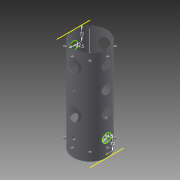
# Autodesk Inventor part: Probe Region Shield
Saved by Autodesk Inventor 2015 (Build 190159000, 159)
## iProperties
Created: 2014-06-23
Part Number: Probe Region Shield
Material: Generic
Document SubType Name: Modeling
Designer: Aki
Density: 1 g/cm^3
Appearance: Default
Author: Aki
Autodesk Inventor part; units mm, degrees
sketch "Sketch1" plane through (0, 0, 0) normal (0, 1, 0) x (-1, 0, 0)
  circle A0 centre (0, 0) radius 84.5
  circle A1 centre (0, 0) radius 85.5
  dimension "d0" = 169
  dimension "d1" = 171
  constraints: 2 centre point, 2 coincident
  measures "d0" diameter of A0
  measures "d1" diameter of A1
extrude "Extrusion1" add sketch "Sketch1" along normal blind 466.5 and the other way blind 15.989
ref_plane "Work Plane1" through (85.5, 0, 0) normal (1, 0, 0) x (0, 1, 0)
ref_plane "Work Plane2" through (-85.5, 0, 0) normal (1, 0, 0) x (0, 1, 0)
sketch "Sketch2" plane through (85.5, 0, 0) normal (1, 0, 0) x (0, 1, 0)
  circle A0 centre (394.5, 0) radius 23.25
  line L0 (466.5, -85.5) -> (466.5, 85.5) projected
  line L1 (-15.989, 85.5) -> (-15.989, -85.5) projected
  point P0 (0, 0)
  dimension "d9" = 46.5
  dimension "d12" = 72
  constraints: 1 centre point, 1 other
  measures "d9" diameter of A0
  measures "d12" distance from line of L0 A0.centre
hole "Hole1" at (85.5, 394.5, 0) direction (-1, 0, 0) diameter 46.5 end through all
sketch "Sketch3" plane through (85.5, 0, 0) normal (1, 0, 0) x (0, 1, 0)
  circle A0 centre (72, 0) radius 23.25
  line L0 (-15.989, 85.5) -> (-15.989, -85.5) projected
  point P0 (0, 0)
  dimension "d21" = 46.5
  dimension "d60" = 72
  constraints: 1 centre point, 1 other
  measures "d21" diameter of A0
  measures "d60" distance of A0.centre point (0, 0)
hole "Hole2" at (85.5, 72, 0) direction (-1, 0, 0) diameter 46.5 end through all
sketch "Sketch4" plane through (85.5, 0, 0) normal (1, 0, 0) x (0, 1, 0)
  circle A0 centre (179.5, 0) radius 23.25
  line L0 (-15.989, 85.5) -> (-15.989, -85.5) projected
  point P0 (0, 0)
  dimension "d30" = 46.5
  dimension "d61" = 179.5
  constraints: 1 centre point, 1 other
  measures "d30" diameter of A0
  measures "d61" distance of A0.centre point (0, 0)
hole "Hole3" at (85.5, 179.5, 0) direction (-1, 0, 0) diameter 46.5 end through all
sketch "Sketch5" plane through (85.5, 0, 0) normal (1, 0, 0) x (0, 1, 0)
  circle A0 centre (287, 0) radius 23.25
  line L0 (-15.989, 85.5) -> (-15.989, -85.5) projected
  point P0 (0, 0)
  dimension "d39" = 46.5
  dimension "d62" = 287
  constraints: 1 centre point, 1 other
  measures "d39" diameter of A0
  measures "d62" distance of A0.centre point (0, 0)
hole "Hole4" at (85.5, 287, 0) direction (-1, 0, 0) diameter 46.5 end through all
sketch "Sketch6" plane through (85.5, 0, 0) normal (1, 0, 0) x (0, 1, 0)
  circle A0 centre (72, 0) radius 22.25
  line L0 (-15.989, 85.5) -> (-15.989, -85.5) projected
  point P0 (0, 0)
  dimension "d48" = 44.5
  dimension "d63" = 72
  constraints: 1 centre point, 1 other
  measures "d48" diameter of A0
  measures "d63" distance of point (0, 0) A0.centre
ref_plane "Work Plane4" through (0, 0, -85.5) normal (0, 0, 1) x (1, 0, 0)
sketch "Sketch9" plane through (0, 0, -85.5) normal (0, 0, 1) x (1, 0, 0)
  circle A0 centre (0, 394.5) radius 35.25
  line L0 (85.5, 466.5) -> (-85.5, 466.5) projected
  point P0 (0, 0)
  dimension "d65" = 70.5
  dimension "d68" = 72
  constraints: 1 centre point
  measures "d65" diameter of A0
  measures "d68" distance from line of L0 A0.centre
sketch "Sketch10" plane through (-85.5, 0, 0) normal (1, 0, 0) x (0, 1, 0)
  circle A0 centre (394.5, 0) radius 22.25
  line L0 (466.5, -85.5) -> (466.5, 85.5) projected
  point P0 (0, 0)
  dimension "d66" = 44.5
  dimension "d67" = 72
  constraints: 1 centre point
  measures "d66" diameter of A0
  measures "d67" distance from line of L0 A0.centre
sketch "Sketch11" plane through (0, 0, -85.5) normal (0, 0, 1) x (1, 0, 0)
  circle A0 centre (0, 179.5) radius 35.25
  line L0 (85.5, 466.5) -> (-85.5, 466.5) projected
  point P0 (0, 0)
  dimension "d69" = 70.5
  dimension "d70" = 287
  constraints: 1 centre point
  measures "d69" diameter of A0
  measures "d70" distance from line of L0 A0.centre
sketch "Sketch12" plane through (0, 0, -85.5) normal (0, 0, 1) x (1, 0, 0)
  circle A0 centre (0, 287) radius 9.9
  line L0 (85.5, 466.5) -> (-85.5, 466.5) projected
  point P0 (0, 0)
  dimension "d71" = 19.8
  dimension "d72" = 179.5
  constraints: 1 centre point
  measures "d71" diameter of A0
  measures "d72" distance from line of L0 A0.centre
sketch "Sketch13" plane through (0, 0, -85.5) normal (0, 0, 1) x (1, 0, 0)
  circle A0 centre (0, 72) radius 9.9
  line L0 (85.5, 466.5) -> (-85.5, 466.5) projected
  point P0 (0, 0)
  dimension "d73" = 19.8
  dimension "d74" = 394.5
  constraints: 1 centre point
  measures "d73" diameter of A0
  measures "d74" distance from line of L0 A0.centre
hole "Hole5" at (0, 394.5, -85.5) direction (0, 0, 1) diameter 70.5 end through all
hole "Hole6" at (0, 179.5, -85.5) direction (0, 0, 1) diameter 70.5 end through all
hole "Hole7" at (0, 287, -85.5) direction (0, 0, 1) diameter 19.8 end through all
hole "Hole8" at (0, 72, -85.5) direction (0, 0, 1) diameter 19.8 end through all
ref_plane "Work Plane5" through (0, 29.7, 0) normal (0, 1, 0) x (-1, 0, 0)
sketch "Sketch15" plane through (0, 29.7, 0) normal (0, 1, 0) x (-1, 0, 0)
  line L0 (-5, 96.5006) -> (5, 96.5006)
  line L1 (5, 96.5006) -> (5, 74.5006)
  line L2 (5, 74.5006) -> (-5, 74.5006)
  line L3 (-5, 74.5006) -> (-5, 96.5006)
  line L4 (-5, 96.5006) -> (5, 74.5006) construction
  line L5 (5, 96.5006) -> (-5, 74.5006) construction
  line L6 (74.4716, 5) -> (96.4716, 5)
  line L7 (96.4716, 5) -> (96.4716, -5)
  line L8 (96.4716, -5) -> (74.4716, -5)
  line L9 (74.4716, -5) -> (74.4716, 5)
  line L10 (74.4716, 5) -> (96.4716, -5) construction
  line L11 (96.4716, 5) -> (74.4716, -5) construction
  line L12 (-5, -74.4994) -> (5, -74.4994)
  line L13 (5, -74.4994) -> (5, -96.4994)
  line L14 (5, -96.4994) -> (-5, -96.4994)
  line L15 (-5, -96.4994) -> (-5, -74.4994)
  line L16 (-5, -74.4994) -> (5, -96.4994) construction
  line L17 (5, -74.4994) -> (-5, -96.4994) construction
  line L18 (-74.5284, 5) -> (-96.5284, 5)
  line L19 (-96.5284, 5) -> (-96.5284, -5)
  line L20 (-96.5284, -5) -> (-74.5284, -5)
  line L21 (-74.5284, -5) -> (-74.5284, 5)
  line L22 (-74.5284, 5) -> (-96.5284, -5) construction
  line L23 (-96.5284, 5) -> (-74.5284, -5) construction
  line L24 (56.215, 49.1439) -> (71.7713, 64.7003)
  line L25 (71.7713, 64.7003) -> (64.7003, 71.7713)
  line L26 (64.7003, 71.7713) -> (49.1439, 56.215)
  line L27 (49.1439, 56.215) -> (56.215, 49.1439)
  circle A0 centre (0, 0) radius 85.5 projected
  line L28 (56.215, 49.1439) -> (64.7003, 71.7713) construction
  line L29 (71.7713, 64.7003) -> (49.1439, 56.215) construction
  line L30 (56.215, 49.1439) -> (78.215, 49.1439) construction
  line L31 (-56.215, 49.1439) -> (-71.7713, 64.7003)
  line L32 (-71.7713, 64.7003) -> (-64.7003, 71.7713)
  line L33 (-64.7003, 71.7713) -> (-49.1439, 56.215)
  line L34 (-49.1439, 56.215) -> (-56.215, 49.1439)
  line L35 (-56.215, 49.1439) -> (-64.7003, 71.7713) construction
  line L36 (-71.7713, 64.7003) -> (-49.1439, 56.215) construction
  line L37 (-56.215, 49.1439) -> (-34.215, 49.1439) construction
  line L38 (-64.7003, -71.7713) -> (-49.1439, -56.215)
  line L39 (-49.1439, -56.215) -> (-56.215, -49.1439)
  line L40 (-56.215, -49.1439) -> (-71.7713, -64.7003)
  line L41 (-71.7713, -64.7003) -> (-64.7003, -71.7713)
  line L42 (-64.7003, -71.7713) -> (-56.215, -49.1439) construction
  line L43 (-49.1439, -56.215) -> (-71.7713, -64.7003) construction
  line L44 (-64.7003, -71.7713) -> (-42.7003, -71.7713) construction
  line L45 (49.1439, -56.215) -> (64.7003, -71.7713)
  line L46 (64.7003, -71.7713) -> (71.7713, -64.7003)
  line L47 (71.7713, -64.7003) -> (56.215, -49.1439)
  line L48 (56.215, -49.1439) -> (49.1439, -56.215)
  line L49 (49.1439, -56.215) -> (71.7713, -64.7003) construction
  line L50 (64.7003, -71.7713) -> (56.215, -49.1439) construction
  line L51 (49.1439, -56.215) -> (71.1439, -56.215) construction
  circle A1 centre (0, 0) radius 85.5
  point P0 (0, 85.5006)
  point P1 (85.4716, 0)
  point P2 (0, -85.4994)
  point P3 (-85.5284, 0)
  point P4 (60.4576, 60.4576)
  point P5 (-60.4576, 60.4576)
  point P6 (-60.4576, -60.4576)
  point P7 (60.4576, -60.4576)
  dimension "d105" = 10
  dimension "d106" = 22
  dimension "d107" = 22
  dimension "d108" = 10
  dimension "d109" = 10
  dimension "d110" = 22
  dimension "d111" = 22
  dimension "d112" = 10
  dimension "d123" = 22
  dimension "d124" = 45
  dimension "d125" = 10
  dimension "d126" = 22
  dimension "d127" = 135
  dimension "d128" = 10
  dimension "d129" = 22
  dimension "d130" = 45
  dimension "d131" = 10
  dimension "d132" = 22
  dimension "d133" = 45
  dimension "d134" = 10
  dimension "d135" = 171
  dimension "d138" = 0
  dimension "d139" = 45
  dimension "d140" = 45
  dimension "d141" = 45
  dimension "d142" = 45
  dimension "d143" = 45
  dimension "d144" = 45
  dimension "d145" = 45
  dimension "d146" = 171
  dimension "d147" = 171
  dimension "d148" = 171
  dimension "d149" = 171
  constraints: 104 end point, 18 parallel, 16 midpoint, 8 horizontal, 8 perpendicular, 4 equal length, 4 point on circle, 1 centre point, 1 coincident
  measures "d105" distance of L1.end L2.end
  measures "d106" distance of L0.end L1.end
  measures "d107" distance of L7.end L8.end
  measures "d108" distance of L6.end L7.end
  measures "d109" distance of L13.end L14.end
  measures "d110" distance of L12.end L13.end
  measures "d111" distance of L20.end L19.end
  measures "d112" distance of L19.end L18.end
  measures "d123" distance of L24.start L24.end
  measures "d124" angle of L30 L24
  measures "d125" distance of L25.end L24.end
  measures "d126" distance of L31.start L31.end
  measures "d127" angle of L37 L31
  measures "d128" distance of L31.end L32.end
  measures "d129" distance of L38.start L38.end
  measures "d130" angle of L44 L38
  measures "d131" distance of L39.end L38.end
  measures "d132" distance of L45.start L45.end
  measures "d133" angle of L45 L51
  measures "d134" distance of L46.end L45.end
  measures "d135" diameter of A1
  measures "d138" vertical distance of point (0, 0) point (85.472, 0)
  measures "d146" distance of point (0, -85.499) point (0, 85.501)
  measures "d147" distance of point (-60.458, -60.458) A0.start
  measures "d148" distance of A0.end point (60.458, -60.458)
  measures "d149" distance of point (85.472, 0) point (-85.528, 0)
extrude "Extrusion3" add sketch "Sketch15" along normal blind 2 contours L0 L1 A0 L3 | A0 L1 L2 L3 | L33 L34 L31 A0 | A0 L31 L32 L33 | A0 L24 L27 L26 | L26 L25 L24 A0 | A0 L20 L19 L18 | L18 L21 L20 A0 | A0 L8 L9 L6 | L6 L7 L8 A0 | L40 L39 L38 A0 | A0 L38 L41 L40 | L47 L46 L45 A0 | A0 L45 L48 L47 | A0 L13 L14 L15 | L15 L12 L13 A0
sketch "Sketch16" plane through (0, 29.7, 0) normal (0, 1, 0) x (-1, 0, 0)
  circle A0 centre (0, 0) radius 85
  dimension "d150" = 170
  constraints: 1 centre point, 1 coincident
  measures "d150" diameter of A0
hole "Hole9" at (0, 29.7, 0) direction (0, 1, 0) diameter 170 end through all
ref_plane "Work Plane6" through (0, 434, 0) normal (0, 1, 0) x (-1, 0, 0)
sketch "Sketch25" plane through (0, 434, 0) normal (0, 1, 0) x (-1, 0, 0)
  line L0 (-4.9993, 74.4997) -> (5.0007, 74.5003)
  line L1 (5.0007, 74.5003) -> (4.9993, 96.5003)
  line L2 (4.9993, 96.5003) -> (-5.0007, 96.4997)
  line L3 (-5.0007, 96.4997) -> (-4.9993, 74.4997)
  circle A0 centre (0, 0) radius 85.5 projected
  line L4 (-4.9993, 74.4997) -> (4.9993, 96.5003) construction
  line L5 (5.0007, 74.5003) -> (-5.0007, 96.4997) construction
  line L6 (-56.215, 49.1439) -> (-49.1439, 56.215)
  line L7 (-49.1439, 56.215) -> (-64.7003, 71.7713)
  line L8 (-64.7003, 71.7713) -> (-71.7713, 64.7003)
  line L9 (-71.7713, 64.7003) -> (-56.215, 49.1439)
  line L10 (-56.215, 49.1439) -> (-64.7003, 71.7713) construction
  line L11 (-49.1439, 56.215) -> (-71.7713, 64.7003) construction
  line L12 (-56.215, 49.1439) -> (-46.215, 49.1439) construction
  line L13 (49.1439, 56.215) -> (64.7003, 71.7713)
  line L14 (64.7003, 71.7713) -> (71.7713, 64.7003)
  line L15 (71.7713, 64.7003) -> (56.215, 49.1439)
  line L16 (56.215, 49.1439) -> (49.1439, 56.215)
  line L17 (49.1439, 56.215) -> (71.7713, 64.7003) construction
  line L18 (64.7003, 71.7713) -> (56.215, 49.1439) construction
  line L19 (49.1439, 56.215) -> (71.1439, 56.215) construction
  line L20 (74.5, -5) -> (96.5, -5)
  line L21 (96.5, -5) -> (96.5, 5)
  line L22 (96.5, 5) -> (74.5, 5)
  line L23 (74.5, 5) -> (74.5, -5)
  line L24 (74.5, -5) -> (96.5, 5) construction
  line L25 (96.5, -5) -> (74.5, 5) construction
  line L26 (96.4716, -5) -> (96.4716, 5) projected
  line L27 (74.5, -5) -> (96.5, -5) construction
  line L28 (-74.5, -5) -> (-96.5, -5)
  line L29 (-96.5, -5) -> (-96.5, 5)
  line L30 (-96.5, 5) -> (-74.5, 5)
  line L31 (-74.5, 5) -> (-74.5, -5)
  line L32 (-74.5, -5) -> (-96.5, 5) construction
  line L33 (-96.5, -5) -> (-74.5, 5) construction
  line L34 (-74.5, -5) -> (-52.5, -5) construction
  circle A1 centre (0, 0) radius 84.5 projected
  line L35 (-5, -74.5) -> (5, -74.5)
  line L36 (5, -74.5) -> (5, -96.5)
  line L37 (5, -96.5) -> (-5, -96.5)
  line L38 (-5, -96.5) -> (-5, -74.5)
  line L39 (-5, -74.5) -> (5, -96.5) construction
  line L40 (5, -74.5) -> (-5, -96.5) construction
  line L41 (-5, -74.5) -> (5, -74.5) construction
  line L42 (49.1439, -56.215) -> (64.7003, -71.7713)
  line L43 (64.7003, -71.7713) -> (71.7713, -64.7003)
  line L44 (71.7713, -64.7003) -> (56.215, -49.1439)
  line L45 (56.215, -49.1439) -> (49.1439, -56.215)
  line L46 (49.1439, -56.215) -> (71.7713, -64.7003) construction
  line L47 (64.7003, -71.7713) -> (56.215, -49.1439) construction
  line L48 (49.1439, -56.215) -> (71.1439, -56.215) construction
  line L49 (-64.7003, -71.7713) -> (-49.1439, -56.215)
  line L50 (-49.1439, -56.215) -> (-56.215, -49.1439)
  line L51 (-56.215, -49.1439) -> (-71.7713, -64.7003)
  line L52 (-71.7713, -64.7003) -> (-64.7003, -71.7713)
  line L53 (-64.7003, -71.7713) -> (-56.215, -49.1439) construction
  line L54 (-49.1439, -56.215) -> (-71.7713, -64.7003) construction
  line L55 (-64.7003, -71.7713) -> (-42.7003, -71.7713) construction
  point P0 (0, 85.5)
  point P1 (-60.4576, 60.4576)
  point P2 (60.4576, 60.4576)
  point P3 (85.5, 0)
  point P4 (-85.5, 0)
  point P5 (0, -85.5)
  point P6 (60.4576, -60.4576)
  point P7 (-60.4576, -60.4576)
  dimension "d0" = 169
  dimension "d236" = 10
  dimension "d237" = 22
  dimension "d238" = 10
  dimension "d239" = 45
  dimension "d240" = 22
  dimension "d241" = 22
  dimension "d242" = 45
  dimension "d243" = 10
  dimension "d244" = 22
  dimension "d245" = 0
  dimension "d246" = 10
  dimension "d247" = 22
  dimension "d248" = 180
  dimension "d249" = 10
  dimension "d253" = 10
  dimension "d254" = 0
  dimension "d255" = 22
  dimension "d256" = 22
  dimension "d257" = 45
  dimension "d258" = 10
  dimension "d259" = 45
  dimension "d260" = 45
  dimension "d261" = 45
  dimension "d262" = 45
  dimension "d264" = 22
  dimension "d265" = 45
  dimension "d266" = 10
  dimension "d267" = 45
  dimension "d268" = 45
  dimension "d269" = 45
  dimension "d319" = 0
  constraints: 110 end point, 16 midpoint, 16 parallel, 10 perpendicular, 9 horizontal, 7 equal length, 9 other
  measures "d236" distance of L0.start L0.end
  measures "d237" distance of L1.end L0.end
  measures "d238" distance of L6.start L6.end
  measures "d239" angle of L12 L6
  measures "d240" distance of L7.end L6.end
  measures "d241" distance of L13.start L13.end
  measures "d242" angle of L19 L13
  measures "d243" distance of L13.end L14.end
  measures "d244" distance of L20.start L20.end
  measures "d245" distance between parallel lines of L20 L27
  measures "d246" distance of L21.end L20.end
  measures "d247" distance of L28.start L28.end
  measures "d248" angle of L28 L34
  measures "d249" distance of L28.end L29.end
  measures "d253" distance of L35.start L35.end
  measures "d254" distance between parallel lines of L35 L41
  measures "d255" distance of L35.end L36.end
  measures "d256" distance of L42.start L42.end
  measures "d257" angle of L42 L48
  measures "d258" distance of L43.end L42.end
  measures "d264" distance of L49.start L49.end
  measures "d265" angle of L55 L49
  measures "d266" distance of L50.end L49.end
  measures "d319" horizontal distance of point (0, 0) point (0, -85.5)
extrude "Extrusion4" add sketch "Sketch25" along normal blind 2 contours L3 A1 L1 L0 | L3 A0 L1 A1 | L3 L2 L1 A0 | A1 L9 A0 L7 | L7 L6 L9 A1 | A1 L15 L16 L13 | L13 A0 L15 A1 | A0 L9 L8 L7 | L13 L14 L15 A0 | A1 L28 A0 L30 | L30 L31 L28 A1 | A0 L28 L29 L30 | L51 L50 L49 A1 | A1 L49 A0 L51 | A0 L49 L52 L51 | L44 A0 L42 A1 | A1 L42 L45 L44 | L38 L35 L36 A1 | A1 L36 A0 L38 | L44 L43 L42 A0 | A0 L36 L37 L38
sketch "Sketch26" plane through (0, 434, 0) normal (0, 1, 0) x (-1, 0, 0)
  circle A0 centre (0, 0) radius 85
  dimension "d272" = 170
  constraints: 1 centre point, 1 coincident
  measures "d272" diameter of A0
hole "Hole18" at (0, 434, 0) direction (0, 1, 0) diameter 170 end through all
sketch "Sketch27" plane through (0, 436, 0) normal (0, 1, 0) x (1, 0, 0)
  circle A0 centre (64.7356, -64.7356) radius 2.15
  line L0 (71.7713, -64.7003) -> (63.8897, -56.8186) projected
  point P0 (0, 0)
  dimension "d280" = 4.3
  dimension "d281" = 91.55
  dimension "d282" = 5
  constraints: 1 centre point
  measures "d280" diameter of A0
  measures "d281" distance of A0.centre point (0, 0)
  measures "d282" distance from line of L0 A0.centre
hole "Hole19" at (64.7356, 436, 64.7356) direction (0, -1, 0) diameter 4.3 end through all
sketch "Sketch28" plane through (0, 436, 0) normal (0, 1, 0) x (1, 0, 0)
  circle A0 centre (91.55, 0) radius 2.15
  point P0 (0, 0)
  dimension "d290" = 4.3
  dimension "d291" = 91.55
  constraints: 1 centre point
  measures "d290" diameter of A0
  measures "d291" distance of point (0, 0) A0.centre
hole "Hole20" at (91.55, 436, 0) direction (0, -1, 0) diameter 4.3 end through all
sketch "Sketch29" plane through (0, 436, 0) normal (0, 1, 0) x (1, 0, 0)
  circle A0 centre (64.7356, 64.7356) radius 2.15
  line L0 (64.7003, 71.7713) -> (56.8186, 63.8897) projected
  point P0 (0, 0)
  dimension "d299" = 4.3
  dimension "d300" = 91.55
  dimension "d301" = 5
  constraints: 1 centre point
  measures "d299" diameter of A0
  measures "d300" distance of A0.centre point (0, 0)
  measures "d301" distance from line of L0 A0.centre
hole "Hole21" at (64.7356, 436, -64.7356) direction (0, -1, 0) diameter 4.3 end through all
sketch "Sketch30" plane through (0, 436, 0) normal (0, 1, 0) x (1, 0, 0)
  circle A0 centre (0.0004, -91.55) radius 2.15
  line L0 (-5, -85.3537) -> (-4.9993, -96.5003) projected
  point P0 (0, 0)
  dimension "d0" = 169
  dimension "d309" = 4.3
  dimension "d310" = 91.55
  dimension "d311" = 5
  constraints: 1 centre point
  measures "d309" diameter of A0
  measures "d310" distance of point (0, 0) A0.centre
  measures "d311" distance from line of L0 A0.centre
hole "Hole22" at (0.0004, 436, 91.55) direction (0, -1, 0) diameter 4.3 end through all
sketch "Sketch31" plane through (0, 436, 0) normal (0, 1, 0) x (1, 0, 0)
  circle A0 centre (-64.7356, -64.7356) radius 2.15
  line L0 (-64.7003, -71.7713) -> (-56.8186, -63.8897) projected
  point P0 (0, 0)
  dimension "d320" = 4.3
  dimension "d321" = 91.55
  dimension "d322" = 5
  constraints: 1 centre point
  measures "d320" diameter of A0
  measures "d321" distance of A0.centre point (0, 0)
  measures "d322" distance from line of L0 A0.centre
hole "Hole23" at (-64.7356, 436, 64.7356) direction (0, -1, 0) diameter 4.3 end through all
sketch "Sketch32" plane through (0, 31.7, 0) normal (0, 1, 0) x (1, 0, 0)
  circle A0 centre (-91.55, 0) radius 2.15
  point P0 (0, 0)
  dimension "d330" = 4.3
  dimension "d331" = 91.55
  constraints: 1 centre point
  measures "d330" diameter of A0
  measures "d331" distance of A0.centre point (0, 0)
hole "Hole24" at (-91.55, 31.7, 0) direction (0, -1, 0) diameter 4.3 end through all
sketch "Sketch33" plane through (0, 436, 0) normal (0, 1, 0) x (1, 0, 0)
  circle A0 centre (-64.7356, 64.7356) radius 2.15
  line L0 (-56.8186, 63.8897) -> (-64.7003, 71.7713) projected
  point P0 (0, 0)
  dimension "d339" = 4.3
  dimension "d340" = 91.55
  dimension "d341" = 5
  constraints: 1 centre point
  measures "d339" diameter of A0
  measures "d340" distance of point (0, 0) A0.centre
  measures "d341" distance from line of L0 A0.centre
hole "Hole25" at (-64.7356, 436, -64.7356) direction (0, -1, 0) diameter 4.3 end through all
sketch "Sketch34" plane through (0, 436, 0) normal (0, 1, 0) x (1, 0, 0)
  circle A0 centre (0, 91.55) radius 2.15
  point P0 (0, 0)
  dimension "d349" = 4.3
  dimension "d350" = 91.55
  constraints: 1 centre point
  measures "d349" diameter of A0
  measures "d350" distance of A0.centre point (0, 0)
hole "Hole26" at (0, 436, -91.55) direction (0, -1, 0) diameter 4.3 end through all
body "Solid1"
